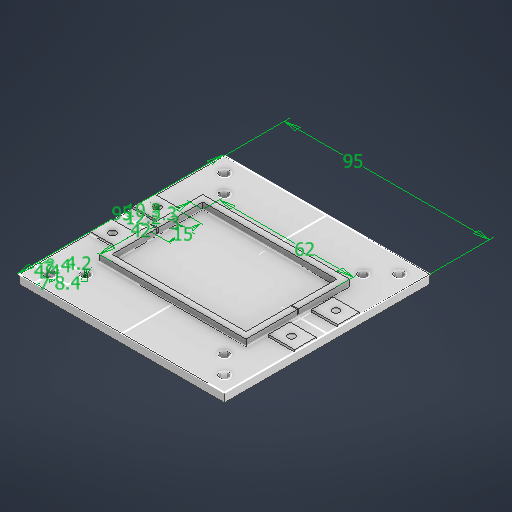
# Autodesk Inventor part: Molde grande 643FBR 1mm
Saved by Autodesk Inventor 2026.1 (Build 301233000, 233)
## iProperties
Created: 2025-11-18
Part Number: Molde grande 643FBR 1mm
Material: Genérico
Document SubType Name: Modeling
Designer: Laboratorio_sensores
Density: 1 g/cm^3
Appearance: Valor por defecto
Author: Laboratorio_sensores
Autodesk Inventor part; units mm, degrees
ref_plane "YZ Plane" through (0, 0, 0) normal (1, 0, 0) x (0, 1, 0)
ref_plane "XZ Plane" through (0, 0, 0) normal (0, 1, 0) x (-1, 0, 0)
ref_plane "XY Plane" through (0, 0, 0) normal (0, 0, 1) x (1, 0, 0)
sketch "Boceto1" plane through (0, 0, 0) normal (0, 1, 0) x (-1, 0, 0)
  line L0 (0, 0) -> (95, 0)
  line L1 (95, 0) -> (95, -95)
  line L2 (95, -95) -> (0, -95)
  line L3 (0, -95) -> (0, 0)
  line L4 (78.5, -26.5) -> (16.5, -26.5)
  line L5 (16.5, -26.5) -> (16.5, -68.5)
  line L6 (16.5, -68.5) -> (78.5, -68.5)
  line L7 (78.5, -68.5) -> (78.5, -26.5)
  line L8 (47.5, -26.5) -> (47.5, 0)
  line L9 (78.5, -47.5) -> (95, -47.5)
  line L10 (47.5, -68.5) -> (47.5, -95)
  line L11 (16.5, -47.5) -> (0, -47.5)
  line L12 (81.5, -23.5) -> (13.5, -23.5)
  line L13 (13.5, -23.5) -> (13.5, -71.5)
  line L14 (13.5, -71.5) -> (81.5, -71.5)
  line L15 (81.5, -71.5) -> (81.5, -23.5)
  line L16 (95, 0) -> (88, 0)
  line L17 (88, 0) -> (88, -7)
  line L18 (88, -7) -> (95, -7)
  line L19 (95, -7) -> (95, 0)
  circle A0 centre (88, -7) radius 2.2
  circle A1 centre (88, -88) radius 2.2
  circle A2 centre (7, -7) radius 2.2
  circle A3 centre (7, -88) radius 2.2
  line L20 (95, -47.5) -> (82.8, -47.5)
  line L21 (82.8, -47.5) -> (82.8, -62.5)
  line L22 (82.8, -62.5) -> (95, -62.5)
  line L23 (82.8, -47.5) -> (82.8, -32.5)
  line L24 (82.8, -32.5) -> (95, -32.5)
  line L25 (88.9, -47.5) -> (88.9, -57.8)
  circle A4 centre (88.9, -57.8) radius 1.65
  circle A5 centre (88.9, -37.2) radius 1.65
  line L26 (12.2, -47.5) -> (12.2, -62.5)
  line L27 (12.2, -62.5) -> (0, -62.5)
  line L28 (12.2, -47.5) -> (12.2, -32.5)
  line L29 (12.2, -32.5) -> (0, -32.5)
  circle A6 centre (6.1, -57.8) radius 1.65
  circle A7 centre (6.1, -37.2) radius 1.65
  line L30 (88, -7) -> (79.6, -7)
  line L31 (88, -7) -> (88, -15.4)
  line L32 (88, -7) -> (79.6, -7)
  line L33 (79.6, -7) -> (79.6, -15.4)
  line L34 (79.6, -15.4) -> (88, -15.4)
  line L35 (88, -15.4) -> (88, -7)
  circle A8 centre (79.6, -15.4) radius 2.1
  circle A9 centre (79.6, -79.6) radius 2.1
  circle A10 centre (15.4, -15.4) radius 2.1
  circle A11 centre (15.4, -79.6) radius 2.1
  point P0 (47.5, -23.5)
  point P1 (47.5, -71.5)
  dimension "d0" = 95
  dimension "d1" = 95
  dimension "d2" = 42
  dimension "d3" = 62
  dimension "d4" = 3
  dimension "d5" = 7
  dimension "d6" = 7
  dimension "d7" = 4.4
  dimension "d10" = 12.2
  dimension "d11" = 15
  dimension "d12" = 10.3
  dimension "d13" = 3.3
  dimension "d29" = 8.4
  dimension "d30" = 8.4
  dimension "d31" = 4.2
  constraints: 72 end point, 16 symmetric about line, 12 centre point, 11 parallel, 11 perpendicular, 9 midpoint, 4 horizontal, 3 coincident, 3 vertical, 2 point on line, 12 other
  measures "d0" distance of L0.end L1.end
  measures "d1" distance of L1.end L2.end
  measures "d2" distance of L6.end L4.start
  measures "d3" distance of L5.end L6.end
  measures "d4" distance between parallel lines of L15 L7
  measures "d5" distance of L16.end L17.end
  measures "d6" distance of L17.end L18.end
  measures "d7" diameter of A0
  measures "d10" distance of L9.end L20.end
  measures "d11" distance of L20.end L21.end
  measures "d12" distance of L25.start L25.end
  measures "d13" diameter of A4
  measures "d29" distance of L30.start L30.end
  measures "d30" distance of L30.start L31.end
  measures "d31" diameter of A8
extrude "Extrusión1" add sketch "Boceto1" against normal blind 4 contours L0 L8 L12 L13 L11 L28 L29 L3 | L0 L17 A0 L30 L33 A8 L34 L31 L18 L1 L24 L23 L9 L15 L12 L8 | L29 L28 L11 L3 | L0 L1 L18 A0 L17 | L12 L15 L9 L7 L4 L8 | L8 L4 L5 L11 L13 L12 | L11 L26 L27 L3 | L4 L7 L6 L5 | L27 L26 L11 L13 L14 L10 L2 L3 | A0 L31 L34 A8 L33 L30 | L15 L14 L10 L6 L7 L9 | L9 L21 L22 L1 L2 L10 L14 L15 | L11 L5 L6 L10 L14 L13 | L1 L9 L23 L24 | L9 L1 L22 L21 | A8 L34 L33 | L33 L34 A8 | A9 | A10 | A11
extrude "Extrusión2" add sketch "Boceto1" along normal blind 3 contours L12 L15 L9 L7 L4 L8 | L8 L4 L5 L11 L13 L12 | L15 L14 L10 L6 L7 L9 | L11 L5 L6 L10 L14 L13
sketch "Boceto2" plane through (0, 3, 0) normal (0, 1, 0) x (1, 0, 0)
  line L0 (-16.5, 47.5) -> (0, 47.5) projected
  line L1 (-47.5, 68.5) -> (-47.5, 95) projected
  line L2 (-13.5, 23.5) -> (-13.5, 71.5) projected
  line L3 (-16.5, 68.5) -> (-16.5, 26.5) projected
  line L4 (-13.5, 47.25) -> (-16.5, 47.25)
  line L5 (-16.5, 47.25) -> (-16.5, 47.75)
  line L6 (-16.5, 47.75) -> (-13.5, 47.75)
  line L7 (-13.5, 47.75) -> (-13.5, 47.25)
  line L8 (-81.5, 23.5) -> (-81.5, 71.5)
  line L9 (-78.5, 68.5) -> (-78.5, 26.5)
  line L10 (-81.5, 47.25) -> (-78.5, 47.25)
  line L11 (-78.5, 47.75) -> (-81.5, 47.75)
  point P0 (0, 0)
  dimension "d16" = 0.5
  dimension "d17" = 0.25
  constraints: 16 end point, 8 symmetric about line, 4 point on line, 2 parallel, 1 horizontal, 1 perpendicular
  measures "d16" distance between parallel lines of L4 L6
  measures "d17" distance between parallel lines of L0 L6
extrude "Extrusión3" cut sketch "Boceto2" against normal blind 2
extrude "Extrusión4" add sketch "Boceto1" along normal blind 1 contours L29 L28 L11 L3 | L11 L26 L27 L3 | L1 L9 L23 L24 | L9 L1 L22 L21
sketch "Boceto3" plane through (0, 1, 0) normal (0, 1, 0) x (1, 0, 0)
  line L0 (-16.5, 47.5) -> (0, 47.5) projected
  line L1 (-12.2, 62.5) -> (-12.2, 32.5) projected
  line L2 (0, 32.5) -> (0, 62.5) projected
  line L3 (-12.2, 42.5) -> (0, 42.5)
  line L4 (0, 42.5) -> (0, 52.5)
  line L5 (0, 52.5) -> (-12.2, 52.5)
  line L6 (-12.2, 52.5) -> (-12.2, 42.5)
  line L7 (-47.5, 68.5) -> (-47.5, 95) projected
  line L8 (-82.8, 62.5) -> (-82.8, 32.5)
  line L9 (-95, 32.5) -> (-95, 62.5)
  line L10 (-82.8, 42.5) -> (-95, 42.5)
  line L11 (-95, 52.5) -> (-82.8, 52.5)
  point P0 (0, 0)
  point P1 (0, 42.5)
  dimension "d22" = 5
  dimension "d23" = 5
  constraints: 16 end point, 8 symmetric about line, 4 point on line, 2 parallel, 1 horizontal, 1 perpendicular
  measures "d22" distance between parallel lines of L3 L0
  measures "d23" distance between parallel lines of L5 L0
extrude "Extrusión5" cut sketch "Boceto3" against normal blind 1
sketch "Boceto4" plane through (0, -4, 0) normal (0, -1, 0) x (1, 0, 0)
  circle A0 centre (-6.1, -37.2) radius 1.65 projected
  line L0 (-2.9823, -37.2) -> (-4.5412, -39.9)
  line L1 (-4.5412, -39.9) -> (-7.6588, -39.9)
  line L2 (-7.6588, -39.9) -> (-9.2177, -37.2)
  line L3 (-9.2177, -37.2) -> (-7.6588, -34.5)
  line L4 (-7.6588, -34.5) -> (-4.5412, -34.5)
  line L5 (-4.5412, -34.5) -> (-2.9823, -37.2)
  line L6 (-16.5, -47.5) -> (0, -47.5) projected
  line L7 (-47.5, -68.5) -> (-47.5, -95) projected
  line L8 (-2.9823, -57.8) -> (-4.5412, -55.1)
  line L9 (-4.5412, -55.1) -> (-7.6588, -55.1)
  line L10 (-7.6588, -55.1) -> (-9.2177, -57.8)
  line L11 (-9.2177, -57.8) -> (-7.6588, -60.5)
  line L12 (-7.6588, -60.5) -> (-4.5412, -60.5)
  line L13 (-4.5412, -60.5) -> (-2.9823, -57.8)
  line L14 (-92.0177, -37.2) -> (-90.4588, -39.9)
  line L15 (-90.4588, -39.9) -> (-87.3412, -39.9)
  line L16 (-87.3412, -39.9) -> (-85.7823, -37.2)
  line L17 (-85.7823, -37.2) -> (-87.3412, -34.5)
  line L18 (-87.3412, -34.5) -> (-90.4588, -34.5)
  line L19 (-90.4588, -34.5) -> (-92.0177, -37.2)
  line L20 (-90.4588, -60.5) -> (-92.0177, -57.8)
  line L21 (-92.0177, -57.8) -> (-90.4588, -55.1)
  line L22 (-90.4588, -55.1) -> (-87.3412, -55.1)
  line L23 (-87.3412, -55.1) -> (-85.7823, -57.8)
  line L24 (-85.7823, -57.8) -> (-87.3412, -60.5)
  line L25 (-87.3412, -60.5) -> (-90.4588, -60.5)
  point P0 (0, 0)
  point P1 (-6.1, -57.8)
  point P2 (-6.1, -39.9)
  point P3 (-6.1, -34.5)
  point P4 (-88.9, -39.9)
  dimension "d26" = 5.4
  constraints: 48 end point, 19 symmetric about line, 2 midpoint, 1 coincident, 13 other
  measures "d26" distance of point (-6.1, -39.9) point (-6.1, -34.5)
extrude "Extrusión6" cut sketch "Boceto4" against normal blind 2.5 contours A0 | L0 L1 L2 L3 L4 L5 | L13 L12 L11 L10 L9 L8 | L19 L18 L17 L16 L15 L14 | L20 L21 L22 L23 L24 L25
extrude "Extrusión7" cut sketch "Boceto1" against normal blind 5 contours A8 L34 L33 | L33 L34 A8 | A9 | A10 | A11
